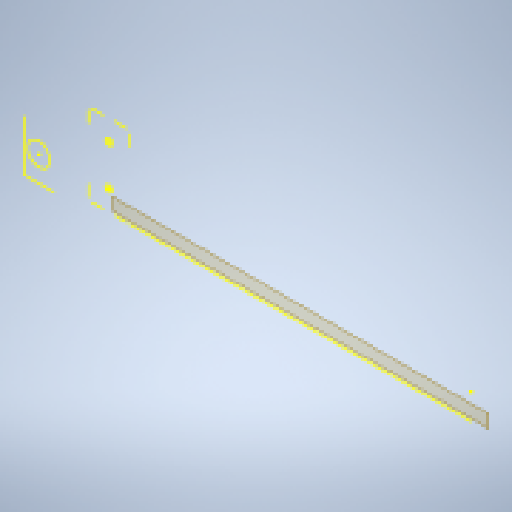
# Autodesk Inventor part: 6MM_ENDPLATE_FIXEDSIDE
Saved by Autodesk Inventor 2025.2 (Build 292293000, 293)
## iProperties
Created: 2026-02-06
Part Number: 6MM_ENDPLATE_FIXEDSIDE
Material: Generic
Document SubType Name: Modeling
Designer: composite
Density: 1 g/cm^3
Appearance: Default
Author: composite
Autodesk Inventor part; units mm, degrees
ref_plane "YZ Plane" through (0, 0, 0) normal (1, 0, 0) x (0, 1, 0)
ref_plane "XZ Plane" through (0, 0, 0) normal (0, 1, 0) x (-1, 0, 0)
ref_plane "XY Plane" through (0, 0, 0) normal (0, 0, 1) x (1, 0, 0)
ref_plane "Work Plane1" through (0, -22.46, 0) normal (0, 0, 1) x (1, 0, 0)
sketch "Sketch1" plane through (0, -22.46, 0) normal (0, 0, 1) x (1, 0, 0)
  circle A0 centre (-356.5, 56.83) radius 3.4 projected
  circle A1 centre (-356.5, 16.83) radius 3.4 projected
  line L0 (-336.5, 62.3996) -> (-336.5, 73.66) projected
  line L1 (-339.6594, 76.83) -> (-350.9175, 76.83) projected
  line L2 (-376.5, 73.8874) -> (-376.5, 62.627) projected
  line L3 (-376.5, 73.8874) -> (-376.5, 62.627) projected
  line L4 (-362.0696, 76.83) -> (-373.33, 76.83) projected
  line L5 (0, -3.17) -> (-336.5, -3.17) projected
  line L6 (-350.9175, -3.17) -> (-339.6594, -3.17) projected
  line L7 (-373.33, -3.17) -> (-362.0696, -3.17) projected
  line L8 (-376.5, 11.033) -> (-376.5, -0.2274) projected
  line L9 (-440.5, -13.17) -> (-410.5, -13.17) projected
  line L10 (-440.5, 36.83) -> (-440.5, -13.17) projected
  circle A2 centre (-425.5, 11.83) radius 11 projected
  point P0 (0, 22.46)
sketch "Sketch2" plane through (0, -22.46, 0) normal (0, 0, 1) x (1, 0, 0)
  circle A0 centre (-321.5, 16.83) radius 2.75
  circle A1 centre (-296.5, 16.83) radius 2.75
  line L0 (-336.5, 62.3996) -> (-336.5, 73.66) projected
  line L1 (0, -3.17) -> (-336.5, -3.17) construction
  circle A2 centre (-425.5, 11.83) radius 11 projected
  circle A3 centre (-425.5, 11.83) radius 21 construction
  circle A4 centre (-425.5, 11.83) radius 33.333 construction
  circle A5 centre (-440.3492, 26.6792) radius 2.25
  circle A6 centre (-449.07, 35.4) radius 2.5
  circle A7 centre (-440.3492, -3.0192) radius 2.25
  circle A8 centre (-410.6508, -3.0192) radius 2.25
  circle A9 centre (-410.6508, 26.6792) radius 2.25
  circle A10 centre (-449.07, -11.74) radius 2.5
  circle A11 centre (-401.93, -11.74) radius 2.5
  circle A12 centre (-401.93, 35.4) radius 2.5
  line L2 (-339.6594, 76.83) -> (-350.9175, 76.83) construction
  line L3 (-362.0696, 76.83) -> (-373.33, 76.83) construction
  line L4 (-376.5, 73.8874) -> (-376.5, 62.627) projected
  line L5 (-350.9175, -3.17) -> (-339.6594, -3.17) construction
  line L6 (-373.33, -3.17) -> (-362.0696, -3.17) construction
  line L7 (-376.5, 11.033) -> (-376.5, -0.2274) construction
  line L8 (-373.33, 76.83) -> (-376.5, 76.83) construction
  line L9 (-376.5, 76.83) -> (-376.5, 73.8874) construction
  line L10 (-336.5, 73.66) -> (-336.5, 76.83) construction
  line L11 (-336.5, 76.83) -> (-339.6594, 76.83) construction
  line L12 (-376.5, -0.2274) -> (-376.5, -3.17) construction
  line L13 (-376.5, -3.17) -> (-336.5, -3.17) construction
  line L14 (-395.8, -17.87) -> (-455.2, -17.87) construction
  line L15 (-455.2, -17.87) -> (-455.2, 41.53) construction
  line L16 (-455.2, 41.53) -> (-395.8, 41.53) construction
  line L17 (-395.8, 41.53) -> (-395.8, -17.87) construction
  line L18 (-395.8, -17.87) -> (-455.2, 41.53) construction
  line L19 (-455.2, -17.87) -> (-395.8, 41.53) construction
  line L20 (-336.5, 76.83) -> (-286.5, 36.83)
  line L21 (-286.5, 36.83) -> (-286.5, -3.17)
  line L22 (-286.5, -3.17) -> (-376.5, -3.17)
  line L23 (-376.5, -3.17) -> (-395.8, -17.87)
  line L24 (-455.2, -17.87) -> (-395.8, -17.87)
  line L25 (-455.2, -17.87) -> (-455.2, 41.53)
  line L26 (-455.2, 41.53) -> (-376.5, 76.83)
  line L27 (-336.5, 76.83) -> (-376.5, 76.83)
  circle A13 centre (-356.5, 56.83) radius 4.5
  circle A14 centre (-356.5, 16.83) radius 4.5
  point P0 (0, 22.46)
  point P1 (-336.5, 68.0298)
  dimension "d5" = 42
  dimension "d0" = 5.5
  dimension "d1" = 5.5
  dimension "d2" = 25
  dimension "d3" = 15
  dimension "d4" = 20
  dimension "d6" = 5
  dimension "d7" = 4.5
  dimension "d10" = 360
  dimension "d14" = 360
  dimension "d16" = 47.14
  dimension "d17" = 59.4
  dimension "d18" = 59.4
  dimension "d21" = 40
  dimension "d22" = 10
  dimension "d26" = 9
  dimension "d27" = 9
  constraints: 40 end point, 12 centre point, 5 perpendicular, 4 coincident, 3 horizontal, 3 midpoint, 3 parallel, 2 collinear, 2 point on line, 2 vertical alignment, 1 horizontal alignment, 1 vertical, 24 other
  measures "d0" diameter of A0
  measures "d1" diameter of A1
  measures "d2" distance of A1.centre A0.centre
  measures "d3" horizontal distance of A0.centre point (-336.5, 68.03)
  measures "d4" distance from line of A0.centre L1
  measures "d6" diameter of A6
  measures "d7" diameter of A5
  measures "d16" distance of A12.centre A6.centre
  measures "d17" distance of L15.end L16.end
  measures "d18" distance of L14.end L15.end
  measures "d21" distance of L20.end L21.end
  measures "d22" distance from line of A1.centre L21
  measures "d26" diameter of A13
  measures "d27" diameter of A14
extrude "Extrusion1" add sketch "Sketch2" along normal blind 6
fillet "Fillet1" radius 5 8 edges at (-376.5, 54.37, 3) (-336.5, 54.37, 3) (-286.5, 14.37, 3) (-286.5, -25.63, 3) (-376.5, -25.63, 3) (-395.8, -40.33, 3) (-455.2, -40.33, 3) (-455.2, 19.07, 3)
equation "\"d18\" = d17"
equation "\"d27\" = d26"
body "Solid1"
